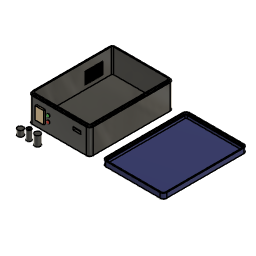
IEB-assembly v4 (Autodesk Fusion 360 archive; units mm, degrees)
design "Caixa_IEB"
Autodesk Fusion 360 part; units mm, degrees
sketch "Sketch1" plane through (0, 0, 0) normal (0, 0, 1) x (1, 0, 0)
  line L0 (2, 0) -> (98, 0)
  line L1 (100, -2) -> (100, -138)
  line L2 (98, -140) -> (2, -140)
  line L3 (0, -138) -> (0, -2)
  arc A0 (2, 0) -> (0, -2) centre (2, -2) ccw
  arc A1 (100, -2) -> (98, 0) centre (98, -2) ccw
  arc A2 (98, -140) -> (100, -138) centre (98, -138) ccw
  arc A3 (0, -138) -> (2, -140) centre (2, -138) ccw
  arc A4 (102, -2) -> (98, 2) centre (98, -2) ccw
  line L4 (2, 2) -> (98, 2)
  arc A5 (2, 2) -> (-2, -2) centre (2, -2) ccw
  line L5 (-2, -138) -> (-2, -2)
  arc A6 (-2, -138) -> (2, -142) centre (2, -138) ccw
  line L6 (98, -142) -> (2, -142)
  arc A7 (98, -142) -> (102, -138) centre (98, -138) ccw
  line L7 (102, -2) -> (102, -138)
  arc A8 (104, -2) -> (98, 4) centre (98, -2) ccw
  line L8 (2, 4) -> (98, 4)
  arc A9 (2, 4) -> (-4, -2) centre (2, -2) ccw
  line L9 (-4, -138) -> (-4, -2)
  arc A10 (-4, -138) -> (2, -144) centre (2, -138) ccw
  line L10 (98, -144) -> (2, -144)
  arc A11 (98, -144) -> (104, -138) centre (98, -138) ccw
  line L11 (104, -2) -> (104, -138)
  arc A12 (102.2, -2) -> (98, 2.2) centre (98, -2) ccw
  line L12 (2, 2.2) -> (98, 2.2)
  arc A13 (2, 2.2) -> (-2.2, -2) centre (2, -2) ccw
  line L13 (-2.2, -138) -> (-2.2, -2)
  arc A14 (-2.2, -138) -> (2, -142.2) centre (2, -138) ccw
  line L14 (98, -142.2) -> (2, -142.2)
  arc A15 (98, -142.2) -> (102.2, -138) centre (98, -138) ccw
  line L15 (102.2, -2) -> (102.2, -138)
  point P0 (100, 0)
  point P1 (0, -140)
  dimension "d1" = 140
  dimension "d2" = 100
  dimension "d3" = 2
  dimension "d4" = -2
  dimension "d5" = -4
  dimension "d6" = -2.2
  constraint horizontal L0
  constraint vertical L1
  constraint horizontal L2
  constraint vertical L3
  constraint coincident origin L0
  constraint coincident origin L3
  constraint tangent L0 A0
  constraint tangent L3 A0
  constraint coincident P0 L0
  constraint coincident P0 L1
  constraint tangent L0 A1
  constraint tangent L1 A1
  constraint equal A0 A1
  constraint tangent L1 A2
  constraint tangent L2 A2
  constraint equal A0 A2
  constraint coincident P1 L2
  constraint coincident P1 L3
  constraint tangent L2 A3
  constraint tangent L3 A3
  constraint equal A0 A3
  measures "d1" distance of origin P1
  measures "d2" distance of origin P0
  measures "d3" radius of A0
  measures "d4" distance of A1
  measures "d5" distance of A1
extrude "Extrude1" add sketch "Sketch1" against normal blind 5 contours L0 L1 L2 L3 A0 A1 A2 A3 | A4 L4 A5 L5 A6 L6 A7 L7 | A8 L8 A9 L9 A10 L10 A11 L11 | A12 L12 A13 L13 A14 L14 A15 L15 makes body 1
extrude "Extrude2" add sketch "Sketch1" along normal blind 42.5 contours A4 L4 A5 L5 A6 L6 A7 L7 bodies 1
extrude "Extrude3" add sketch "Sketch1" along normal up to surface (40 mm away) contours A8 L8 A9 L9 A10 L10 A11 L11 | A12 L12 A13 L13 A14 L14 A15 L15 bodies 1
copy_body "Body->Comp1" bodies 1 removing the originals makes body 2 in component "Component"
extrude "Extrude1'" add sketch "Sketch1" along normal blind 10 from surface at 40 separate body contours A8 L8 A9 L9 A10 L10 A11 L11 makes body 3 in component "Component'"
extrude "Extrude2'" add sketch "Sketch1" against normal blind 7.5 from surface at 50 contours A4 L4 A5 L5 A6 L6 A7 L7 | A12 L12 A13 L13 A14 L14 A15 L15 bodies 3 in component "Component'"
extrude "Extrude3'" add sketch "Sketch1" against normal blind 3 from surface at 50 contours L0 L1 L2 L3 A0 A1 A2 A3 bodies 3 in component "Component'"
fillet "Fillet1" radius 1.5 8 edges at (50, -144, -5) (-2.2426, -142.2426, -5) (-4, -70, -5) (-2.2426, 2.2426, -5) (50, 4, -5) (102.2426, 2.2426, -5) (104, -70, -5) (102.2426, -142.2426, -5) on bodies 2 in component "Component"
fillet "Fillet1'" radius 1.5 8 edges at (50, 4, 50) (-2.2426, 2.2426, 50) (-4, -70, 50) (-2.2426, -142.2426, 50) (50, -144, 50) (102.2426, -142.2426, 50) (104, -70, 50) (102.2426, 2.2426, 50) on bodies 3 in component "Component'"
sketch "Sketch2" plane through (0, -144, 0) normal (0, -1, 0) x (1, 0, 0)
  line L0 (2, -3.5) -> (98, -3.5)
  line L1 (98, -3.5) -> (98, 40)
  line L2 (98, 40) -> (2, 40)
  line L3 (2, 40) -> (2, -3.5)
  line L4 (12, 29) -> (24.2, 29)
  line L5 (24.2, 29) -> (24.2, 10)
  line L6 (24.2, 10) -> (12, 10)
  line L7 (12, 10) -> (12, 29)
  line L8 (0, 0) -> (0, 42.5)
  line L9 (0, 42.5) -> (0, 0)
  line L10 (2, -5) -> (98, -5)
  line L11 (74.7, 29) -> (88, 29)
  line L12 (88, 29) -> (88, 23.8)
  line L13 (88, 23.8) -> (74.7, 23.8)
  line L14 (74.7, 23.8) -> (74.7, 29)
  line L15 (74.7, 29) -> (24.2, 29) construction
  line L16 (100, 0) -> (100, 42.5) construction
  line L17 (100, 42.5) -> (100, 0) construction
  line L18 (24.2, 19.5) -> (31.2, 19.5) construction
  line L19 (31.2, 19.5) -> (31.2, 24.5) construction
  line L20 (31.2, 19.5) -> (31.2, 14.5) construction
  circle A0 centre (31.2, 24.5) radius 2.5
  circle A1 centre (31.2, 14.5) radius 2.5
  dimension "d27" = 12.2
  dimension "d28" = 19
  dimension "d29" = 12
  dimension "d30" = 15
  dimension "d31" = 5.2
  dimension "d32" = 13.3
  dimension "d45" = 11
  dimension "d47" = 12
  dimension "d78" = 5
  dimension "d79" = 10
  dimension "d80" = 7
  constraint horizontal L4
  constraint vertical L5
  constraint horizontal L6
  constraint vertical L7
  constraint horizontal L11
  constraint vertical L12
  constraint horizontal L13
  constraint vertical L14
  constraint horizontal L15
  constraint midpoint L5 L18.start
  constraint perpendicular L5 L18
  constraint perpendicular L18 L19
  constraint perpendicular L18 L20
  constraint equal L19 L20
  constraint coincident L19.end A0.centre
  constraint coincident L20.end A1.centre
  constraint equal A0 A1
  measures "d27" distance of L4.start L4.end
  measures "d28" distance of L4.start L6.end
  measures "d29" distance of L7 L9
  measures "d30" distance of L6 L10
  measures "d31" distance of L11.start L13.end
  measures "d32" distance of L11.start L11.end
  measures "d45" distance of L2 L4
  measures "d47" distance of L12 L16
  measures "d78" diameter of A0
  measures "d79" distance of L19.end L20.end
  measures "d80" distance of L18.start L18.end
extrude "Extrude1''" cut sketch "Sketch2" against normal blind 20 contours L4 L5 L6 L7 | L11 L12 L13 L14 | A0 | A1 bodies 2 in component "Component"
sketch "Sketch3" plane through (0, 0, 0) normal (0, 0, 1) x (-1, 0, 0)
  line L0 (0, 2) -> (0, 138)
  arc A0 (0, 138) -> (-2, 140) centre (-2, 138) ccw
  line L1 (-2, 140) -> (-98, 140)
  arc A1 (-98, 140) -> (-100, 138) centre (-98, 138) ccw
  line L2 (-100, 138) -> (-100, 2)
  arc A2 (-100, 2) -> (-98, 0) centre (-98, 2) ccw
  line L3 (-98, 0) -> (-2, 0)
  arc A3 (-2, 0) -> (0, 2) centre (-2, 2) ccw
  circle A4 centre (-71, 13) radius 4
  circle A5 centre (-71, 13) radius 2
  line L4 (-71, 13) -> (-71, 131) construction
  circle A6 centre (-71, 131) radius 4
  circle A7 centre (-71, 131) radius 2
  dimension "d36" = 8
  dimension "d37" = 4
  dimension "d38" = 118
  dimension "d39" = 29
  dimension "d40" = 13
  constraint concentric A4 A5
  constraint coincident A4.centre A5.centre
  constraint vertical L4
  constraint coincident L4.end A6.centre
  constraint equal A4 A6
  constraint equal A5 A7
  measures "d36" diameter of A4
  measures "d37" diameter of A5
  measures "d38" distance of A4.centre L4.end
  measures "d39" distance of L2 L4
  measures "d40" distance of L3 A4.centre
extrude "Extrude2''" cut sketch "Sketch3" against normal blind 25 contours A5 | A7 bodies 2 in component "Component"
extrude "Extrude3''" cut sketch "Sketch3" against normal blind 2.5 contours A4 | A6 bodies 2 in component "Component"
sketch "Sketch4" plane through (0, 0, 0) normal (0, 0, 1) x (1, 0, 0)
  circle A0 centre (12, -174) radius 5
  line L0 (12, -174) -> (27, -174) construction
  line L1 (27, -174) -> (42, -174) construction
  circle A1 centre (27, -174) radius 4
  circle A2 centre (27, -174) radius 2
  circle A3 centre (42, -174) radius 5
  line L2 (98, -144) -> (2, -144)
  dimension "d48" = 10
  dimension "d49" = 15
  dimension "d50" = 15
  dimension "d51" = 8
  dimension "d52" = 4
  dimension "d53" = 10
  dimension "d62" = 30
  dimension "d63" = 10
  constraint coincident A0.centre L0.start
  constraint horizontal L0
  constraint parallel L0 L1
  constraint coincident L0.end L1.start
  constraint coincident L1.end A3.centre
  measures "d48" diameter of A0
  measures "d49" distance of A0.centre L0.end
  measures "d50" distance of L0.end L1.end
  measures "d51" diameter of A1
  measures "d52" diameter of A2
  measures "d53" diameter of A3
  measures "d62" distance of L0 L2
  measures "d63" horizontal distance of A0.centre L2.end
extrude "Extrude4" add sketch "Sketch4" along normal blind 17.2 separate body contours A3 makes body 4
extrude "Extrude5" add sketch "Sketch4" along normal blind 3 separate body contours A2 makes body 5
extrude "Extrude6" add sketch "Sketch4" along normal blind 17 contours A1 bodies 5
extrude "Extrude7" add sketch "Sketch4" along normal blind 10 separate body contours A0 makes body 6
sketch "Sketch5" plane through (0, 0, -5) normal (0, 0, -1) x (1, 0, 0)
  circle A0 centre (71, 13) radius 2
  circle A1 centre (71, 131) radius 2
  line L0 (98, 142.5) -> (2, 142.5)
  arc A2 (2, 142.5) -> (-2.5, 138) centre (2, 138) ccw
  line L1 (-2.5, 138) -> (-2.5, 2)
  arc A3 (-2.5, 2) -> (2, -2.5) centre (2, 2) ccw
  line L2 (2, -2.5) -> (98, -2.5)
  arc A4 (98, -2.5) -> (102.5, 2) centre (98, 2) ccw
  line L3 (102.5, 2) -> (102.5, 138)
  arc A5 (102.5, 138) -> (98, 142.5) centre (98, 138) ccw
  line L4 (7.5, 132.5) -> (7.5, 7.5) construction
  line L5 (7.5, 7.5) -> (92.5, 7.5) construction
  line L6 (92.5, 7.5) -> (92.5, 132.5) construction
  line L7 (92.5, 132.5) -> (7.5, 132.5) construction
  circle A6 centre (7.5, 132.5) radius 5.15
  circle A7 centre (92.5, 132.5) radius 5.15
  circle A8 centre (92.5, 7.5) radius 5.15
  circle A9 centre (7.5, 7.5) radius 5.15
  point P0 (50, 70)
  dimension "d64" = -10
  dimension "d65" = 10.3
  constraint coincident L4.start L7.end
  constraint coincident L6.end L7.start
  constraint coincident L5.end L6.start
  constraint coincident L4.end L5.start
  constraint equal A6 A7
  constraint equal A6 A9
  constraint equal A6 A8
  measures "d65" diameter of A6
extrude "Extrude4'" cut sketch "Sketch5" against normal blind 0.6 contours A6 | A7 | A8 | A9 bodies 2 in component "Component"
sketch "Sketch6" plane through (-4, 0, 0) normal (-1, 0, 0) x (0, -1, 0)
  line L0 (2, -3.5) -> (138, -3.5)
  line L1 (138, -3.5) -> (138, 40)
  line L2 (138, 40) -> (2, 40)
  line L3 (2, 40) -> (2, -3.5)
  line L4 (17, 28) -> (18, 28)
  line L5 (18, 28) -> (18, 7)
  line L6 (18, 7) -> (17, 7)
  line L7 (17, 7) -> (17, 28)
  line L8 (-4, 40) -> (-4, -3.5)
  line L9 (20, 28) -> (20, 7)
  line L10 (20, 7) -> (19, 7)
  line L11 (19, 28) -> (20, 28)
  line L12 (19, 7) -> (19, 28)
  line L13 (22, 28) -> (22, 7)
  line L14 (22, 7) -> (21, 7)
  line L15 (21, 28) -> (22, 28)
  line L16 (21, 7) -> (21, 28)
  line L17 (24, 28) -> (24, 7)
  line L18 (24, 7) -> (23, 7)
  line L19 (23, 28) -> (24, 28)
  line L20 (23, 7) -> (23, 28)
  line L21 (26, 28) -> (26, 7)
  line L22 (26, 7) -> (25, 7)
  line L23 (25, 28) -> (26, 28)
  line L24 (25, 7) -> (25, 28)
  line L25 (28, 28) -> (28, 7)
  line L26 (28, 7) -> (27, 7)
  line L27 (27, 28) -> (28, 28)
  line L28 (27, 7) -> (27, 28)
  line L29 (30, 28) -> (30, 7)
  line L30 (30, 7) -> (29, 7)
  line L31 (29, 28) -> (30, 28)
  line L32 (29, 7) -> (29, 28)
  line L33 (32, 28) -> (32, 7)
  line L34 (32, 7) -> (31, 7)
  line L35 (31, 28) -> (32, 28)
  line L36 (31, 7) -> (31, 28)
  line L37 (34, 28) -> (34, 7)
  line L38 (34, 7) -> (33, 7)
  line L39 (33, 28) -> (34, 28)
  line L40 (33, 7) -> (33, 28)
  line L41 (36, 28) -> (36, 7)
  line L42 (36, 7) -> (35, 7)
  line L43 (35, 28) -> (36, 28)
  line L44 (35, 7) -> (35, 28)
  line L45 (38, 28) -> (38, 7)
  line L46 (38, 7) -> (37, 7)
  line L47 (37, 28) -> (38, 28)
  line L48 (37, 7) -> (37, 28)
  line L49 (40, 28) -> (40, 7)
  line L50 (40, 7) -> (39, 7)
  line L51 (39, 28) -> (40, 28)
  line L52 (39, 7) -> (39, 28)
  line L53 (42, 28) -> (42, 7)
  line L54 (42, 7) -> (41, 7)
  line L55 (41, 28) -> (42, 28)
  line L56 (41, 7) -> (41, 28)
  line L57 (44, 28) -> (44, 7)
  line L58 (44, 7) -> (43, 7)
  line L59 (43, 28) -> (44, 28)
  line L60 (43, 7) -> (43, 28)
  line L61 (46, 28) -> (46, 7)
  line L62 (46, 7) -> (45, 7)
  line L63 (45, 28) -> (46, 28)
  line L64 (45, 7) -> (45, 28)
  line L65 (48, 28) -> (48, 7)
  line L66 (48, 7) -> (47, 7)
  line L67 (47, 28) -> (48, 28)
  line L68 (47, 7) -> (47, 28)
  dimension "d68" = 12
  dimension "d69" = 21
  dimension "d70" = 1
  dimension "d71" = 21
  dimension "d74" = 2
  dimension "d75" = 0
  constraint horizontal L4
  constraint vertical L5
  constraint horizontal L6
  constraint vertical L7
  measures "d68" distance of L2 L4
  measures "d69" distance of L7 L8
  measures "d70" distance of L5 L7
  measures "d71" distance of L4.start L6.end
extrude "Extrude5'" cut sketch "Sketch6" against normal blind 10 contours L4 L5 L6 L7 | L9 L10 L11 L12 | L13 L14 L15 L16 | L17 L18 L19 L20 | L21 L22 L23 L24 | L25 L26 L27 L28 | L29 L30 L31 L32 | L33 L34 L35 L36 | L37 L38 L39 L40 | L41 L42 L43 L44 | L45 L46 L47 L48 | L49 L50 L51 L52 | L53 L54 L55 L56 | L57 L58 L59 L60 | L61 L62 L63 L64 | L65 L66 L67 L68 bodies 2 in component "Component"
move_body "Move1" bodies 3 to x (-1, 0, 0) y (0, 1, 0) z (0, 0, -1) at (230, 0, 45) in component "Component'"
sketch "Sketch7" plane through (0, -144, 0) normal (0, -1, 0) x (1, 0, 0)
  line L0 (88, 29) -> (88, 23.8)
  line L1 (88, 23.8) -> (74.7, 23.8)
  line L2 (74.7, 23.8) -> (74.7, 29)
  line L3 (74.7, 29) -> (88, 29)
  circle A0 centre (31.2, 24.5) radius 2.5
  line L4 (24.2, 29) -> (24.2, 10)
  line L5 (24.2, 10) -> (12, 10)
  line L6 (12, 10) -> (12, 29)
  line L7 (12, 29) -> (24.2, 29)
  circle A1 centre (31.2, 14.5) radius 2.5
  line L8 (2, -3.5) -> (98, -3.5)
  line L9 (98, -3.5) -> (98, 40)
  line L10 (98, 40) -> (2, 40)
  line L11 (2, 40) -> (2, -3.5)
  line L12 (25.7, 8.5) -> (10.5, 8.5)
  line L13 (10.5, 8.5) -> (10.5, 30.5)
  line L14 (10.5, 30.5) -> (25.7, 30.5)
  line L15 (25.7, 30.5) -> (25.7, 8.5)
  dimension "d81" = -1.5
extrude "Extrude1'''" add sketch "Sketch7" along normal blind 3 separate body contours A0 | L4 L5 L6 L7 | A1 | L12 L13 L14 L15 makes body 7 at (33.6876, -145, 24.2511) makes body 8 at (33.6876, -145, 14.2511) makes body 9 at (20.6333, -144, 15.8333) in component "Component''"
fillet "Fillet1''" radius 2.5 2 edges at (28.8692, -147, 23.596) (28.8692, -147, 13.596) on bodies 7 8 in component "Component''"
component "Component" placed x (1, 0, 0) y (0, 1, 0) z (0, 0, 1) at (0, 0, 0)
component "Component'" placed x (1, 0, 0) y (0, 1, 0) z (0, 0, 1) at (0, 0, 0)
component "Component''" placed x (1, 0, 0) y (0, 1, 0) z (0, 0, 1) at (0, 0, 0)
named bodies: "Base"

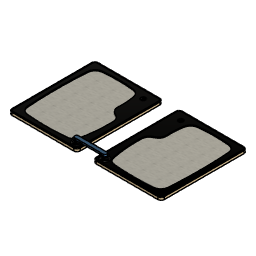
design "Maos IEB"
Autodesk Fusion 360 part; units mm, degrees
sketch "Sketch1" plane through (0, 0, 0) normal (0, 0, 1) x (1, 0, 0)
  line L0 (-228.8074, -5) -> (-35, -5)
  line L1 (-25, -15) -> (-25, -265)
  line L2 (-35, -275) -> (-228.8074, -275)
  line L3 (-238.8074, -265) -> (-238.8074, -15)
  arc A0 (-218.8074, -25) -> (-218.8074, -255) centre (1101.1926, -140) ccw
  arc A1 (-83.5994, -25) -> (-218.8074, -25) centre (-151.2034, -479.5304) ccw
  arc A2 (-78.8074, -116.436) -> (-83.5994, -25) centre (-288.0073, -81.5561) ccw
  arc A3 (-45, -125.4947) -> (-78.8074, -116.436) centre (-81.4607, -193.9531) ccw
  arc A4 (-218.8074, -255) -> (-56.3302, -255) centre (-137.5688, 402.4707) ccw
  arc A5 (-56.3302, -255) -> (-45, -125.4947) centre (-469.0669, -153.6419) ccw
  line L4 (-218.8074, -255) -> (-218.8074, -25) construction
  line L5 (-218.8074, -25) -> (-83.5994, -25) construction
  line L6 (-78.8074, -116.436) -> (-83.5994, -25) construction
  line L7 (-78.8074, -116.436) -> (-45, -125.4947) construction
  line L8 (-45, -125.4947) -> (-56.3302, -255) construction
  line L9 (-56.3302, -255) -> (-218.8074, -255) construction
  line L10 (-223.8074, -140) -> (-218.8074, -140) construction
  line L11 (-151.2034, -20) -> (-151.2034, -25) construction
  line L12 (-76.2102, -70.4563) -> (-81.2034, -70.718) construction
  line L13 (-50.6651, -190.2473) -> (-45.6841, -190.6831) construction
  line L14 (-137.5688, -255) -> (-137.5688, -260) construction
  line L15 (-61.3861, -119.0335) -> (-61.9037, -120.9654) construction
  arc A6 (-228.8074, -5) -> (-238.8074, -15) centre (-228.8074, -15) ccw
  arc A7 (-25, -15) -> (-35, -5) centre (-35, -15) ccw
  arc A8 (-35, -275) -> (-25, -265) centre (-35, -265) ccw
  arc A9 (-238.8074, -265) -> (-228.8074, -275) centre (-228.8074, -265) ccw
  line L16 (0, 0) -> (0, -43.4181) construction
  arc A10 (-28, -15) -> (-35, -8) centre (-35, -15) ccw
  line L17 (-228.8074, -8) -> (-35, -8)
  arc A11 (-228.8074, -8) -> (-235.8074, -15) centre (-228.8074, -15) ccw
  line L18 (-235.8074, -265) -> (-235.8074, -15)
  arc A12 (-235.8074, -265) -> (-228.8074, -272) centre (-228.8074, -265) ccw
  line L19 (-35, -272) -> (-228.8074, -272)
  arc A13 (-35, -272) -> (-28, -265) centre (-35, -265) ccw
  line L20 (-28, -15) -> (-28, -265)
  line L21 (-235.5074, -265) -> (-235.5074, -15)
  arc A14 (-228.8074, -8.3) -> (-235.5074, -15) centre (-228.8074, -15) ccw
  line L22 (-228.8074, -8.3) -> (-35, -8.3)
  arc A15 (-28.3, -15) -> (-35, -8.3) centre (-35, -15) ccw
  line L23 (-28.3, -15) -> (-28.3, -265)
  arc A16 (-35, -271.7) -> (-28.3, -265) centre (-35, -265) ccw
  line L24 (-35, -271.7) -> (-228.8074, -271.7)
  arc A17 (-235.5074, -265) -> (-228.8074, -271.7) centre (-228.8074, -265) ccw
  dimension "d1" = 95
  dimension "d2" = 100
  dimension "d3" = 93
  dimension "d4" = 20
  dimension "d5" = 20
  dimension "d6" = 5
  dimension "d7" = 2
  dimension "d8" = 5
  dimension "d9" = 20
  dimension "d10" = 20
  dimension "d11" = 10
  dimension "d12" = 3
  dimension "d13" = -3.3
  dimension "d25" = 25
  dimension "d26" = 5
  dimension "d61" = 140
  dimension "d62" = 230
  dimension "d63" = 130
  dimension "d64" = 35
  constraint horizontal L0
  constraint vertical L1
  constraint horizontal L2
  constraint vertical L3
  constraint horizontal L9
  constraint horizontal L5
  constraint vertical L4
  constraint midpoint A0 L10.start
  constraint midpoint L4 L10.end
  constraint midpoint A1 L11.start
  constraint midpoint L5 L11.end
  constraint midpoint A2 L12.start
  constraint midpoint L6 L12.end
  constraint midpoint L8 L13.start
  constraint midpoint A5 L13.end
  constraint midpoint L9 L14.start
  constraint midpoint A4 L14.end
  constraint midpoint A3 L15.start
  constraint midpoint L7 L15.end
  constraint equal L10 L11
  constraint equal L11 L12
  constraint equal L10 L14
  constraint tangent L0 A6
  constraint tangent L3 A6
  constraint tangent L0 A7
  constraint tangent L1 A7
  constraint equal A6 A7
  constraint tangent L1 A8
  constraint tangent L2 A8
  constraint equal A6 A8
  constraint tangent L2 A9
  constraint tangent L3 A9
  constraint equal A6 A9
  constraint coincident L16.start origin
  constraint vertical L16
  measures "d1" angle of L8 L9
  measures "d2" angle of L7 L8
  measures "d3" angle of L5 L6
  measures "d4" distance of L0 L5
  measures "d5" distance of L3 L4
  measures "d6" distance of L10.start L10.end
  measures "d7" distance of L15.start L15.end
  measures "d8" distance of L13.start L13.end
  measures "d9" distance of L2 L9
  measures "d10" distance of L1 A3.start
  measures "d11" radius of A6
  measures "d25" distance of L1 L16
  measures "d26" distance of L16.start L0
  measures "d61" distance of A2.start L4
  measures "d62" distance of L5 L9
  measures "d63" distance of A3.start A4.end
  measures "d64" distance of A2.start A3.start
extrude "Extrude1" add sketch "Sketch1" against normal blind 3 contours L0 L1 L2 L3 A6 A7 A8 A9 | A0 A1 A2 A3 A4 A5 | A10 L17 A11 L18 A12 L19 A13 L20 | L21 A14 L22 A15 L23 A16 L24 A17 makes body 1
extrude "Extrude2" add sketch "Sketch1" along normal blind 5 contours L0 L1 L2 L3 A6 A7 A8 A9 bodies 1
extrude "Extrude1'" add sketch "Sketch1" along normal blind 3 separate body contours L21 A14 L22 A15 L23 A16 L24 A17 makes body 2 in component "Component"
fillet "Fillet1" radius 25 6 edges at (-218.8074, -25, 1.5) (-83.5994, -25, 1.5) (-78.8074, -116.436, 1.5) (-45, -125.4947, 1.5) (-56.3302, -255, 1.5) (-218.8074, -255, 1.5) on bodies 2 in component "Component"
sketch "Sketch2" plane through (0, 0, 3) normal (0, 0, 1) x (-1, 0, 0)
  line L0 (28.3, 265) -> (28.3, 15)
  line L1 (35, 8.3) -> (228.8074, 8.3)
  line L2 (235.5074, 15) -> (235.5074, 265)
  line L3 (228.8074, 271.7) -> (35, 271.7)
  arc A0 (76.3086, 94.3954) -> (60.2868, 119.2587) centre (51.3544, 95.9089) ccw
  arc A1 (44.2286, 141.9189) -> (60.2868, 119.2587) centre (69.2191, 142.6085) ccw
  arc A2 (52.3227, 237.0041) -> (44.2286, 141.9189) centre (469.0669, 153.6419) ccw
  arc A3 (74.4553, 256.9867) -> (52.3227, 237.0041) centre (76.837, 232.1004) ccw
  arc A4 (197.7951, 257.2567) -> (74.4553, 256.9867) centre (137.5688, -402.4707) ccw
  arc A5 (220.4592, 234.1364) -> (197.7951, 257.2567) centre (195.5223, 232.3602) ccw
  arc A6 (220.4318, 45.4799) -> (220.4592, 234.1364) centre (-1101.1926, 140) ccw
  arc A7 (198.0437, 22.3935) -> (220.4318, 45.4799) centre (195.4955, 47.2633) ccw
  arc A8 (101.3189, 22.7156) -> (198.0437, 22.3935) centre (151.2034, 479.5304) ccw
  arc A9 (79.4488, 43.0261) -> (101.3189, 22.7156) centre (104.0328, 47.5679) ccw
  arc A10 (76.3086, 94.3954) -> (79.4488, 43.0261) centre (288.0073, 81.5561) ccw
  circle A11 centre (59, 33.3) radius 7.5
  circle A12 centre (-59, 33.3) radius 7.5
  line L4 (-59, 33.3) -> (59, 33.3) construction
  line L5 (0, 33.3) -> (0, 0)
  line L6 (61.3094, 29.3) -> (63.6188, 33.3)
  line L7 (63.6188, 33.3) -> (61.3094, 37.3)
  line L8 (61.3094, 37.3) -> (56.6906, 37.3)
  line L9 (56.6906, 37.3) -> (54.3812, 33.3)
  line L10 (54.3812, 33.3) -> (56.6906, 29.3)
  line L11 (56.6906, 29.3) -> (61.3094, 29.3)
  circle A13 centre (44.3, 256.7) radius 6
  circle A14 centre (-63.1507, 257.4382) radius 46.1789
  circle A15 centre (44.3, 256.7) radius 10
  line L12 (0, 33.3) -> (0, 410.3453)
  circle A16 centre (44.3, 256.7) radius 5.8
  arc A17 (228.8074, 8.3) -> (235.5074, 15) centre (228.8074, 15) ccw
  arc A18 (235.5074, 265) -> (228.8074, 271.7) centre (228.8074, 265) ccw
  arc A19 (35, 271.7) -> (28.3, 265) centre (35, 265) ccw
  arc A20 (28.3, 15) -> (35, 8.3) centre (35, 15) ccw
  point P0 (59, 33.3)
  dimension "d29" = 25
  dimension "d30" = 118
  dimension "d31" = 15
  dimension "d35" = 8
  dimension "d38" = 4
  dimension "d39" = 12
  dimension "d44" = 16
  dimension "d45" = 0.2
  dimension "d65" = 15
  constraint coincident A12.centre L4.start
  constraint coincident P0 A11.centre
  constraint horizontal L4
  constraint equal A11 A12
  constraint midpoint L4 L5.start
  constraint perpendicular L4 L5
  constraint coincident L5.end origin
  constraint concentric A13 A15
  constraint perpendicular L4 L12
  constraint concentric A15 A16
  constraint horizontal L11
  measures "d29" distance of L1 L4
  measures "d30" distance of A12.centre P0
  measures "d31" diameter of A11
  measures "d35" distance of L7 L10
  measures "d38" distance of A13 A15
  measures "d39" diameter of A13
  measures "d44" distance of L0 A13.centre
  measures "d45" distance of A13 A16
  measures "d65" distance of L3 A13.centre
extrude "Extrude2'" cut sketch "Sketch2" against normal blind 20 contours A11 | L6 L7 L8 L9 L10 L11 bodies 2 in component "Component"
extrude "Extrude3" cut sketch "Sketch2" against normal blind 8 contours L6 L7 L8 L9 L10 L11 bodies 1
extrude "Extrude3'" add sketch "Sketch2" along normal blind 10 contours A15 bodies 2 in component "Component"
fillet "Fillet2" radius 4 1 edges at (-34.9767, -260.3162, 3) on bodies 2 in component "Component"
sketch "Sketch3" plane through (0, 0, 13) normal (0, 0, 1) x (-1, 0, 0)
  circle A0 centre (44.3, 256.7) radius 6
  circle A1 centre (44.3, 256.7) radius 10
  line L0 (0, 0) -> (0, -76.6678)
  line L1 (0, -76.6678) -> (0, 297.2205)
  circle A2 centre (44.3, 256.7) radius 5.8
  line L2 (44.4656, 250.9024) -> (0, 250.9024)
  line L3 (44.3, 262.5) -> (0, 262.5)
  dimension "d46" = -0.2
  constraint coincident L0.start origin
  constraint vertical L0
  constraint parallel L0 L1
  constraint coincident A2 L2.start
  constraint coincident L1 L2.end
  constraint perpendicular L1 L2
  constraint coincident A2 L3.start
  constraint coincident L1 L3.end
  constraint tangent A2 L3
  constraint perpendicular L1 L3
extrude "Extrude4" add sketch "Sketch3" against normal blind 10 from surface at 1 separate body contours A2 L2 picked at (45.9803, 258.1985) makes body 3
extrude "Extrude5" add sketch "Sketch3" along normal blind 5 from surface at 1 contours A0 A2 L2 L3 | A0 A1 L2 L3 | A2 L2 | A1 L1 L2 L3 picked at (39.9251, 252.8072) picked at (35.6491, 256.7025) picked at (45.9803, 258.1985) bodies 3
mirror "Mirror2" about plane through (0, -250.9024, 14) normal (1, 0, 0) of bodies 3 merged
mirror "Mirror3" about plane through (0, 0, 0) normal (1, 0, 0) of bodies 1 makes body 4
mirror "Mirror1" about plane through (0, 0, 0) normal (1, 0, 0) of bodies 2 makes body 5 in component "Component"
move_body "Move1" bodies 3 to x (1, 0, 0) y (0, 1, 0) z (0, 0, 1) at (0, 0, 3)
move_body "Move1'" bodies 2 5 to x (1, 0, 0) y (0, 1, 0) z (0, 0, 1) at (0, 0, 3) in component "Component"
extrude "Extrude6" add 2 faces at (-108.3723, -189.1, 0) (108.3723, -189.1, 0) along direction (0, 0, 1) blind 3 separate body on bodies 1 4 makes body 6 at (-108.3723, -189.1, 0) makes body 7 at (108.3723, -189.1, 0)
component "Component" placed x (1, 0, 0) y (0, 1, 0) z (0, 0, 1) at (0, 0, 0)
